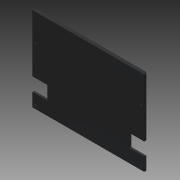
# Autodesk Inventor part: vrchna_platna2
Saved by Autodesk Inventor 2015 (Build 190159000, 159)
## iProperties
Created: 2015-06-11
Part Number: vrchna_platna2
Material: ABS Plastic
Document SubType Name: Modeling
Designer: Jufo
Density: 1 g/cm^3
Appearance: Smooth - White
Author: Jufo
Autodesk Inventor part; units mm, degrees
ref_plane "YZ Plane" through (0, 0, 0) normal (1, 0, 0) x (0, 1, 0)
ref_plane "XZ Plane" through (0, 0, 0) normal (0, 1, 0) x (-1, 0, 0)
ref_plane "XY Plane" through (0, 0, 0) normal (0, 0, 1) x (1, 0, 0)
sketch "Sketch1" plane through (0, 0, 0) normal (0, 1, 0) x (-1, 0, 0)
  line L0 (18.1293, 34.8534) -> (18.1293, -53.1466)
  line L1 (18.1293, -53.1466) -> (40.6293, -53.1466)
  line L2 (40.6293, -53.1466) -> (40.6293, -73.1466)
  line L3 (40.6293, -73.1466) -> (18.1293, -73.1466)
  line L4 (18.1293, -73.1466) -> (18.1293, -93.1466)
  line L5 (18.1293, -93.1466) -> (188.1293, -93.1466)
  line L6 (18.1293, 34.8534) -> (188.1293, 34.8534)
  line L7 (188.1293, 34.8534) -> (188.1293, -52.3568)
  line L8 (188.1293, -52.3568) -> (165.6293, -52.3568)
  line L9 (165.6293, -52.3568) -> (165.6293, -73.0062)
  line L10 (165.6293, -73.0062) -> (188.1293, -73.0062)
  line L11 (188.1293, -73.0062) -> (188.1293, -93.1466)
  point P0 (0, 0)
  dimension "d0" = 88
  dimension "d2" = 22.5
  dimension "d3" = 22.5
  dimension "d4" = 20
  dimension "d5" = 20
  dimension "d6" = 170
  dimension "d64" = 22.5
  dimension "d65" = 22.5
  dimension "d66" = 170
  constraints: 24 end point, 7 perpendicular, 3 parallel, 1 vertical
  measures "d0" distance of L0.start L0.end
  measures "d2" distance of L0.end L1.end
  measures "d3" distance of L2.end L3.end
  measures "d4" distance of L1.end L2.end
  measures "d5" distance of L3.end L4.end
  measures "d6" distance of L4.end L5.end
  measures "d64" distance of L7.end L8.end
  measures "d65" distance of L9.end L10.end
  measures "d66" distance of L0.start L6.end
extrude "Extrusion1" add sketch "Sketch1" along normal blind 3
sketch "Sketch2" plane through (0, 3, 0) normal (0, 1, 0) x (1, 0, 0)
  line L0 (-18.1293, -34.8534) -> (-18.1293, 53.1466) projected
  line L1 (-18.1293, 53.1466) -> (-40.6293, 53.1466) projected
  line L2 (-40.6293, 53.1466) -> (-40.6293, 73.1466) projected
  line L3 (-40.6293, 73.1466) -> (-18.1293, 73.1466) projected
  line L4 (-18.1293, 73.1466) -> (-18.1293, 93.1466) projected
  line L5 (-18.1293, 93.1466) -> (-188.1293, 93.1466) projected
  line L6 (-188.1293, 93.1466) -> (-188.1293, 73.0062) projected
  line L7 (-188.1293, 73.0062) -> (-165.6293, 73.0062) projected
  line L8 (-165.6293, 73.0062) -> (-165.6293, 52.3568) projected
  line L9 (-165.6293, 52.3568) -> (-188.1293, 52.3568) projected
  line L10 (-188.1293, 52.3568) -> (-188.1293, -34.8534) projected
  line L11 (-188.1293, -34.8534) -> (-18.1293, -34.8534) projected
  line L12 (-185.6293, 91.1466) -> (-185.6293, 77.5062)
  line L13 (-185.6293, 77.5062) -> (-159.1293, 77.5062)
  line L14 (-159.1293, 77.5062) -> (-159.1293, 47.8568)
  line L15 (-159.1293, 47.8568) -> (-185.6293, 47.8568)
  line L16 (-185.6293, 47.8568) -> (-185.6293, -34.8534)
  line L17 (-20.6293, 91.1466) -> (-20.6293, 77.6466)
  line L18 (-20.6293, 77.6466) -> (-47.1293, 77.6466)
  line L19 (-47.1293, 77.6466) -> (-47.1293, 48.6466)
  line L20 (-47.1293, 48.6466) -> (-20.6293, 48.6466)
  line L21 (-20.6293, 48.6466) -> (-20.6293, -34.8534)
  line L22 (-185.6293, 91.1466) -> (-20.6293, 91.1466)
  line L23 (-20.6293, -34.8534) -> (-18.1293, -34.8534)
  line L24 (-185.6293, -34.8534) -> (-188.1293, -34.8534)
  point P0 (0, 0)
  dimension "d9" = 6.5
  dimension "d10" = 4.5
  dimension "d11" = 4.5
  dimension "d12" = 2.5
  dimension "d13" = 2.5
  dimension "d57" = 6.5
  dimension "d58" = 4.5
  dimension "d59" = 4.5
  dimension "d60" = 2.5
  dimension "d67" = 2
  constraints: 26 end point, 4 perpendicular, 3 parallel, 1 collinear, 1 point on line
  measures "d9" distance between parallel lines of L14 L8
  measures "d10" distance between parallel lines of L7 L13
  measures "d11" distance between parallel lines of L15 L9
  measures "d12" distance between parallel lines of L10 L16
  measures "d13" distance between parallel lines of L6 L12
  measures "d57" distance between parallel lines of L2 L19
  measures "d58" distance between parallel lines of L18 L3
  measures "d59" distance between parallel lines of L1 L20
  measures "d60" distance between parallel lines of L0 L21
  measures "d67" distance between parallel lines of L22 L5
extrude "Extrusion2" add sketch "Sketch2" along normal blind 2 contours L11 L16 L15 L14 L13 L12 L22 L17 L18 L19 L20 L21
sketch "Sketch3" plane through (0, 5, 0) normal (0, 1, 0) x (1, 0, 0)
  line L0 (-20.6293, -34.8534) -> (-20.6293, 48.6466) projected
  line L1 (-20.6293, 77.6466) -> (-20.6293, 91.1466) projected
  line L2 (-20.6293, 91.1466) -> (-185.6293, 91.1466) projected
  line L3 (-185.6293, 91.1466) -> (-185.6293, 77.5062) projected
  line L4 (-185.6293, -34.8534) -> (-20.6293, -34.8534) projected
  line L5 (-20.6293, 6.8966) -> (-20.6293, 9.8966)
  line L6 (-103.1293, -34.8534) -> (-103.1293, 6.8959)
  line L7 (-185.6293, 91.1466) -> (-185.6293, 85.6466)
  line L8 (-185.6293, 85.6466) -> (-180.1293, 85.6466)
  line L9 (-180.1293, 85.6466) -> (-180.1293, 91.1466)
  line L10 (-20.6293, 91.1466) -> (-26.1293, 91.1466)
  line L11 (-26.1293, 91.1466) -> (-26.1293, 85.6466)
  line L12 (-26.1293, 85.6466) -> (-20.6293, 85.6466)
  circle A0 centre (-23.1293, 88.3966) radius 1.5
  circle A1 centre (-183.1293, 88.6466) radius 1.5
  line L13 (-159.1293, 47.8568) -> (-185.6293, 47.8568) projected
  line L14 (-185.6293, 47.8568) -> (-185.6293, 9.6466)
  line L15 (-185.6293, 9.6466) -> (-180.1293, 9.6466)
  line L16 (-180.1293, 9.6466) -> (-180.1293, 3.6466)
  line L17 (-180.1293, 3.6466) -> (-185.6293, 3.6466)
  line L18 (-185.6293, 3.6466) -> (-185.6293, 9.6466)
  circle A2 centre (-183.1293, 6.6466) radius 1.5
  line L19 (-20.6293, 9.6466) -> (-26.1293, 9.6466)
  line L20 (-26.1293, 9.6466) -> (-26.1293, 3.6466)
  line L21 (-26.1293, 3.6466) -> (-20.6293, 3.6466)
  line L22 (-20.6293, 3.6466) -> (-20.6293, 9.6466)
  circle A3 centre (-23.1293, 6.6466) radius 1.5
  line L23 (-18.1293, 53.1466) -> (-40.6293, 53.1466) projected
  line L24 (-40.6293, 73.1466) -> (-18.1293, 73.1466) projected
  line L25 (-188.1293, 52.3568) -> (-188.1293, -34.8534) projected
  line L26 (-18.1293, 73.1466) -> (-18.1293, 93.1466) projected
  point P0 (0, 0)
  dimension "d23" = 5.5
  dimension "d24" = 5.5
  dimension "d25" = 5.5
  dimension "d26" = 5.5
  dimension "d27" = 3
  dimension "d28" = 3
  dimension "d33" = 6
  dimension "d36" = 3
  dimension "d43" = 5.5
  dimension "d48" = 2.75
  dimension "d49" = 2.5
  dimension "d55" = 5
  dimension "d56" = 2.5
  dimension "d61" = 3
  dimension "d62" = 3
  dimension "d63" = 3
  dimension "d69" = 41.5
  dimension "d72" = 41.5
  constraints: 34 end point, 6 perpendicular, 5 point on line, 5 symmetric about line, 4 centre point, 2 midpoint, 2 parallel, 1 collinear, 1 other
  measures "d23" distance of L2.end L7.end
  measures "d24" distance of L7.end L8.end
  measures "d25" distance of L1.end L10.end
  measures "d26" distance of L10.end L11.end
  measures "d27" diameter of A0
  measures "d28" diameter of A1
  measures "d33" distance of L15.end L16.end
  measures "d36" distance from line of L15 A2.centre
  measures "d43" distance of L16.end L17.end
  measures "d48" distance from line of A0.centre L2
  measures "d49" distance from line of L2 A1.centre
  measures "d55" distance from line of L26 A0.centre
  measures "d56" distance from line of L3 A1.centre
  measures "d61" distance from line of L16 A2.centre
  measures "d62" distance from line of L9 A1.centre
  measures "d63" distance from line of L11 A0.centre
  measures "d69" distance from line of L4 A3.centre
  measures "d72" distance from line of A2.centre L4
extrude "Extrusion4" cut sketch "Sketch3" against normal blind 5 contours A0 | A1 | A2 | A3
equation "\"d3\" = d2"
equation "\"d10\" = d59"
equation "\"d11\" = d59"
equation "\"d12\" = d13"
equation "\"d58\" = d59"
body "Solid1"
